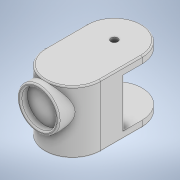
# Autodesk Inventor part: Wirst2
Saved by Autodesk Inventor 2021 (Build 250183000, 183)
## iProperties
Created: 2024-09-30
Part Number: Wirst2
Material: Generic
Document SubType Name: Modeling
Designer: Swoby
Density: 1 g/cm^3
Appearance: Default
Author: Swoby
Autodesk Inventor part; units mm, degrees
ref_plane "YZ Plane" through (0, 0, 0) normal (1, 0, 0) x (0, 1, 0)
ref_plane "XZ Plane" through (0, 0, 0) normal (0, 1, 0) x (-1, 0, 0)
sketch "Sketch1" plane through (0, 0, 0) normal (0, 1, 0) x (-1, 0, 0)
  arc A0 (26.4575, 30) -> (-26.4575, 30) centre (0, 0) ccw construction
  arc A1 (40, 60) -> (-40, 60) centre (0, 60) ccw
  line L0 (0, 100) -> (0, 0) construction
  line L1 (40, 60) -> (40, 0)
  line L2 (-40, 60) -> (-40, 0)
  arc A2 (26.4575, 30) -> (40, 60) centre (0, 60) ccw construction
  arc A3 (40, 0) -> (26.4575, 30) centre (0, 0) ccw construction
  arc A4 (-40, 60) -> (26.4575, 30) centre (0, 60) ccw construction
  arc A5 (-26.4575, 30) -> (-40, 0) centre (0, 0) ccw construction
  arc A6 (-40, 0) -> (40, 0) centre (0, 0) ccw
  circle A7 centre (0, 0) radius 5
  dimension "d0" = 80
  dimension "d1" = 80
  dimension "d2" = 100
  dimension "d3" = 10
  constraints: 18 point on circle, 8 centre point, 6 end point, 4 tangent, 2 coincident, 2 vertical, 1 parallel, 1 point on line
  measures "d0" diameter of A0
  measures "d1" diameter of A1
  measures "d2" distance of point (0, 0) L0.start
  measures "d3" diameter of A7
extrude "Extrusion1" add sketch "Sketch1" along normal mid plane 90
sketch "Sketch2" plane through (0, 0, 0) normal (0, 1, 0) x (-1, 0, 0)
  circle A0 centre (0, 0) radius 5 projected
  circle A1 centre (0, 0) radius 45
  dimension "d6" = 90
  constraints: 1 centre point, 1 coincident
  measures "d6" diameter of A1
extrude "Extrusion2" cut sketch "Sketch2" along normal mid plane 70
fillet "Fillet1" radius 2 10 edges at (40, 0, 20.6155) (-40, 0, 20.6155) (0, 45, -40) (-40, 45, 30) (0, 45, 100) (40, 45, 30) (0, -45, 100) (-40, -45, 30) (0, -45, -40) (40, -45, 30)
ref_plane "Work Plane1" through (40, 0, 60) normal (0, 0, -1) x (0, -1, 0)
sketch "Sketch3" plane through (40, 0, 60) normal (0, 0, -1) x (0, -1, 0)
  circle A0 centre (-13.55, 40) radius 30
  line L0 (0, 40) -> (-13.55, 40)
  dimension "d10" = 60
  dimension "d11" = 13.55
  constraints: 2 end point, 1 centre point, 1 horizontal
  measures "d10" diameter of A0
  measures "d11" distance of L0.start L0.end
extrude "Extrusion3" add sketch "Sketch3" against normal blind 50
sketch "Sketch4" plane through (0, 13.55, 110) normal (0, 0, 1) x (1, 0, 0)
  circle A0 centre (0, 0) radius 30 projected
  circle A1 centre (0, 0) radius 25
  point P0 (0, -13.55)
  dimension "d14" = 50
  constraints: 1 centre point, 1 coincident
  measures "d14" diameter of A1
extrude "Extrusion4" cut sketch "Sketch4" against normal blind 10 contours A1
fillet "Fillet2" radius 2 2 edges at (0, 43.55, 110) (-25, 13.55, 110)
body "Solid1"
